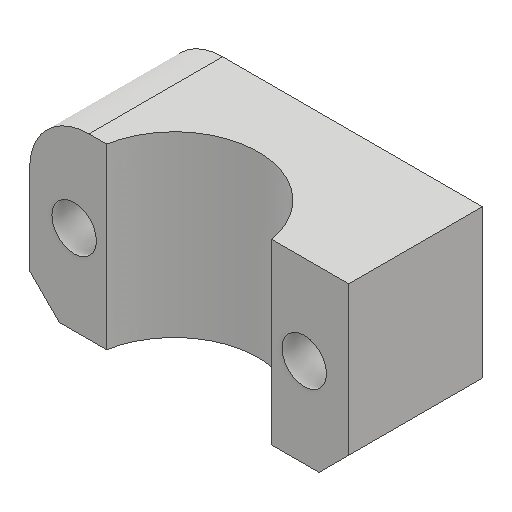
# Autodesk Inventor part: 3DP_ABS_Induction_Sensor_Mounting_Clamp
Saved by Autodesk Inventor 2026.1 (Build 301233000, 233)
## iProperties
Created: 2017-05-27
Part Number: 3DP_ABS_Induction_Sensor_Mounting_Clamp
Material: Ogólny
Document SubType Name: Modeling
Designer: Andrzej
Density: 1 g/cm^3
Appearance: Domyślna
Mass: 1.66103 g
Surface Area: 11.8657 cm^2
Volume: 1.66103 cm^3
Author: Andrzej
Autodesk Inventor part; units mm, degrees
ref_plane "YZ Plane" through (0, 0, 0) normal (1, 0, 0) x (0, 1, 0)
ref_plane "XZ Plane" through (0, 0, 0) normal (0, 1, 0) x (-1, 0, 0)
ref_plane "XY Plane" through (0, 0, 0) normal (0, 0, 1) x (1, 0, 0)
sketch "Szkic1" plane through (0, 0, 0) normal (0, 0, 1) x (1, 0, 0)
  circle A0 centre (0, 0) radius 5.65
  line L0 (-10.75, 1) -> (10.75, 1)
  line L1 (10.75, 1) -> (10.75, 10)
  line L2 (10.75, 10) -> (-10.75, 10)
  line L3 (-10.75, 10) -> (-10.75, 1)
  dimension "d0" = 11.3
  dimension "d1" = 21.5
  dimension "d2" = 10.75
  dimension "d3" = 1
  dimension "d4" = 9
  constraints: 8 end point, 2 parallel, 1 centre point, 1 coincident, 1 horizontal, 1 perpendicular
  measures "d0" diameter of A0
  measures "d1" distance between parallel lines of L1 L3
  measures "d2" distance from line of L3 point (0, 0)
  measures "d3" distance from line of L0 point (0, 0)
  measures "d4" distance between parallel lines of L2 L0
extrude "Wyciągnięcie proste1" add sketch "Szkic1" along normal blind 12 contours L0 A0 | A0 L0 L3 L2 L1 picked at (1.0817, 2.5289)
extrude "Wyciągnięcie proste2" cut sketch "Szkic1" along normal blind 12 contours A0 L0 | L0 A0
sketch "Szkic2" plane through (10.75, 1, 0) normal (0, -1, 0) x (1, 0, 0)
  line L0 (-5.1892, 12) -> (-5.1892, 0) projected
  line L1 (-5.1892, 0) -> (0, 0) projected
  line L2 (0, 0) -> (0, 12) projected
  line L3 (-5.1892, 12) -> (0, 12) projected
  line L4 (-16.3108, 0) -> (-16.3108, 12) projected
  line L5 (-21.5, 12) -> (-16.3108, 12) projected
  line L6 (-21.5, 0) -> (-21.5, 12) projected
  line L7 (-21.5, 0) -> (-16.3108, 0) projected
  point P0 (-10.75, 0)
  point P1 (-3, 6)
  point P2 (-18.5, 6)
  dimension "d9" = 12
  dimension "d10" = 5.1892
  dimension "d11" = 3
  dimension "d12" = 6
  dimension "d13" = 6
  dimension "d14" = 3
  measures "d9" distance of L1.end L2.end
  measures "d10" distance of L0.end L1.end
  measures "d11" distance from line of L2 point (-3, 6)
  measures "d12" distance from line of L1 point (-3, 6)
  measures "d13" distance from line of L7 point (-18.5, 6)
  measures "d14" distance from line of L6 point (-18.5, 6)
hole "Otwór1" at (7.75, 1, 6) at (-7.75, 1, 6) direction (0, 1, 0) diameter 3 end through all
fillet "Zaokrąglenie1" radius 4 1 edges at (-10.75, 5.5, 12)
chamfer "Faza1" distance 2 angle 45 2 edges at (-10.75, 5.5, 0) (10.75, 5.5, 0)
equation "\"d2\" = 0.5 * d1"
equation "\"d12\" = 0.5 * d9"
equation "\"d13\" = d12"
equation "\"d14\" = d11"
